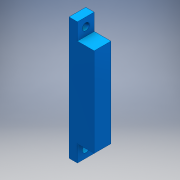
# Autodesk Inventor part: frontBeam
Saved by Autodesk Inventor 2016 (Build 200138000, 138)
## iProperties
Created: 2016-06-14
Part Number: frontBeam
Material: ABS Plastic
Document SubType Name: Modeling
Designer: hesaon
Density: 1.06 g/cm^3
Appearance: Smooth - White
Author: hesaon
Autodesk Inventor part; units mm, degrees
ref_plane "YZ Plane" through (0, 0, 0) normal (1, 0, 0) x (0, 1, 0)
ref_plane "XZ Plane" through (0, 0, 0) normal (0, 1, 0) x (-1, 0, 0)
ref_plane "XY Plane" through (0, 0, 0) normal (0, 0, 1) x (1, 0, 0)
sketch "Sketch1" plane through (0, 0, 0) normal (0, 1, 0) x (-1, 0, 0)
  line L0 (0, 0) -> (10, 0)
  line L1 (10, 0) -> (10, 10)
  line L2 (10, 10) -> (15, 10)
  line L3 (15, 10) -> (15, -63)
  line L4 (15, -63) -> (10, -63)
  line L5 (10, -63) -> (10, -53)
  line L6 (10, -53) -> (0, -53)
  line L7 (0, -53) -> (0, 0)
  dimension "d6" = 53
  dimension "d7" = 73
  dimension "d8" = 10
  dimension "d9" = 5
  dimension "d10" = 10
  constraints: 16 end point, 6 perpendicular, 2 point on line, 1 horizontal
  measures "d6" distance between parallel lines of L0 L6
  measures "d7" distance between parallel lines of L4 L2
  measures "d8" distance between parallel lines of L6 L4
  measures "d9" distance between parallel lines of L5 L3
  measures "d10" distance between parallel lines of L1 L7
extrude "Extrusion1" add sketch "Sketch1" along normal blind 10
hole "Hole1" at (-10, 5, 5) direction (-1, 0, 0) diameter 4.2 end through all
hole "Hole2" at (-10, 5, -58) direction (-1, 0, 0) diameter 4.2 end through all
body "Solid1"
